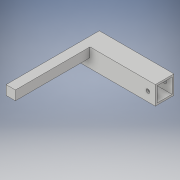
# Autodesk Inventor part: hollowPart
Saved by Autodesk Inventor 2019 (Build 230136000, 136)
## iProperties
Created: 2018-11-15
Part Number: hollowPart
Material: Generic
Document SubType Name: Modeling
Designer: Charlie
Density: 1 g/cm^3
Appearance: Default
Author: Charlie
Autodesk Inventor part; units mm, degrees
ref_plane "YZ Plane" through (0, 0, 0) normal (1, 0, 0) x (0, 1, 0)
ref_plane "XZ Plane" through (0, 0, 0) normal (0, 1, 0) x (-1, 0, 0)
ref_plane "XY Plane" through (0, 0, 0) normal (0, 0, 1) x (1, 0, 0)
sketch "Sketch1" plane through (0, 0, 0) normal (0, 0, 1) x (1, 0, 0)
  line L0 (-25.4, 6.35) -> (25.4, 6.35)
  line L1 (25.4, 6.35) -> (25.4, -6.35)
  line L2 (25.4, -6.35) -> (-25.4, -6.35)
  line L3 (-25.4, -6.35) -> (-25.4, 6.35)
  point P0 (0, 0)
  dimension "d0" = 50.8
  dimension "d1" = 12.7
  dimension "d2" = 25.4
  dimension "d3" = 6.35
  constraints: 8 end point, 2 parallel, 1 horizontal, 1 perpendicular
  measures "d0" distance of L1.end L2.end
  measures "d1" distance between parallel lines of L2 L0
  measures "d2" distance from line of L1 point (0, 0)
  measures "d3" distance from line of L0 point (0, 0)
extrude "Extrusion1" add sketch "Sketch1" along normal blind 12.7
sketch "Sketch2" plane through (25.4, -6.35, 0) normal (1, 0, 0) x (0, 0, -1)
  line L0 (-11.43, 11.43) -> (-1.27, 11.43)
  line L1 (-1.27, 11.43) -> (-1.27, 1.27)
  line L2 (-1.27, 1.27) -> (-11.43, 1.27)
  line L3 (-11.43, 1.27) -> (-11.43, 11.43)
  line L4 (-12.7, 0) -> (-12.7, 12.7) projected
  line L5 (0, 12.7) -> (-12.7, 12.7) projected
  point P0 (0, 6.35)
  dimension "d6" = 10.16
  dimension "d7" = 10.16
  dimension "d8" = 1.27
  dimension "d9" = 1.27
  constraints: 8 end point, 2 parallel, 1 horizontal, 1 perpendicular
  measures "d6" distance between parallel lines of L2 L0
  measures "d7" distance between parallel lines of L1 L3
  measures "d8" distance between parallel lines of L4 L3
  measures "d9" distance between parallel lines of L5 L0
extrude "Extrusion2" cut sketch "Sketch2" against normal blind 49.53
sketch "Sketch3" plane through (0, 0, 12.7) normal (0, 0, 1) x (1, 0, 0)
  line L0 (-25.4, 6.35) -> (-19.05, 6.35)
  line L1 (-19.05, 6.35) -> (-19.05, 0)
  line L2 (-19.05, 0) -> (-25.4, 0)
  line L3 (-25.4, 0) -> (-25.4, 6.35)
  line L4 (-25.4, 6.35) -> (-25.4, -6.35) projected
  line L5 (25.4, 6.35) -> (-25.4, 6.35) projected
  point P0 (0, 0)
  dimension "d12" = 0
  dimension "d13" = 6.35
  dimension "d14" = 0
  dimension "d15" = 6.35
  constraints: 8 end point, 2 parallel, 1 horizontal, 1 perpendicular
  measures "d12" distance between parallel lines of L3 L4
  measures "d13" distance between parallel lines of L3 L1
  measures "d14" distance between parallel lines of L5 L0
  measures "d15" distance between parallel lines of L0 L2
extrude "Extrusion3" add sketch "Sketch3" along normal blind 50.8
sketch "Sketch4" plane through (0, 0, 12.7) normal (0, 0, 1) x (1, 0, 0)
  circle A0 centre (20.32, 0) radius 1.27
  line L0 (25.4, 6.35) -> (-19.05, 6.35) projected
  point P0 (0, 0)
  dimension "d18" = 2.54
  dimension "d19" = 20.32
  dimension "d20" = 6.35
  constraints: 1 centre point
  measures "d18" diameter of A0
  measures "d19" distance of point (0, 0) A0.centre
  measures "d20" distance from line of L0 A0.centre
extrude "Extrusion4" cut sketch "Sketch4" against normal blind 50.8
body "Solid1"
